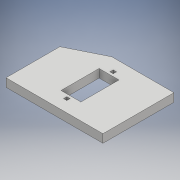
# Autodesk Inventor part: BackHand
Saved by Autodesk Inventor 2018 (Build 220112000, 112)
## iProperties
Created: 2018-02-14
Part Number: BackHand
Material: Générique
Document SubType Name: Modeling
Designer: Thomas
Density: 1 g/cm^3
Appearance: Par défaut
Author: Thomas
Autodesk Inventor part; units mm, degrees
ref_plane "YZ Plane" through (0, 0, 0) normal (1, 0, 0) x (0, 1, 0)
ref_plane "XZ Plane" through (0, 0, 0) normal (0, 1, 0) x (-1, 0, 0)
ref_plane "XY Plane" through (0, 0, 0) normal (0, 0, 1) x (1, 0, 0)
sketch "Esquisse1" plane through (0, 0, 0) normal (0, 0, 1) x (1, 0, 0)
  line L0 (0, 0) -> (0, 32.5)
  line L1 (0, 0) -> (58.5, 0)
  line L2 (58.5, 0) -> (58.5, 42.9)
  line L3 (58.5, 42.9) -> (21, 42.9)
  line L4 (0, 32.5) -> (21, 42.9)
  line L5 (58.5, 42.9) -> (0, 42.9) construction
  line L6 (0, 42.9) -> (0, 0) construction
  line L7 (0, 42.9) -> (58.5, 0) construction
  line L8 (58.5, 42.9) -> (0, 0) construction
  dimension "d0" = 32.5
  dimension "d1" = 58.5
  dimension "d2" = 42.9
  dimension "d3" = 37.5
  constraints: 18 end point, 3 horizontal, 2 vertical, 1 perpendicular
  measures "d0" distance of L0.start L0.end
  measures "d1" distance of L0.start L1.end
  measures "d2" distance of L1.end L2.end
  measures "d3" distance of L2.end L3.end
extrude "Extrusion1" add sketch "Esquisse1" along normal blind 5
sketch "Esquisse2" plane through (0, 0, 5) normal (0, 0, 1) x (1, 0, 0)
  line L0 (23.25, 32.95) -> (35.25, 32.95)
  line L1 (35.25, 32.95) -> (35.25, 9.95)
  line L2 (35.25, 9.95) -> (23.25, 9.95)
  line L3 (23.25, 9.95) -> (23.25, 32.95)
  line L4 (0, 32.5) -> (0, 0) projected
  line L5 (58.5, 42.9) -> (21, 42.9) projected
  line L6 (28.25, 36.45) -> (30.25, 36.45)
  line L7 (30.25, 36.45) -> (30.25, 34.45)
  line L8 (30.25, 34.45) -> (28.25, 34.45)
  line L9 (28.25, 34.45) -> (28.25, 36.45)
  line L10 (28.25, 8.45) -> (30.25, 8.45)
  line L11 (30.25, 8.45) -> (30.25, 6.45)
  line L12 (30.25, 6.45) -> (28.25, 6.45)
  line L13 (28.25, 6.45) -> (28.25, 8.45)
  dimension "d6" = 23
  dimension "d7" = 12
  dimension "d8" = 23.25
  dimension "d9" = 9.95
  dimension "d10" = 2
  dimension "d11" = 2
  dimension "d12" = 2
  dimension "d13" = 2
  dimension "d14" = 1.5
  dimension "d15" = 1.5
  dimension "d16" = 5
  dimension "d17" = 5
  constraints: 24 end point, 6 parallel, 3 horizontal, 3 perpendicular
  measures "d6" distance of L0.end L1.end
  measures "d7" distance of L1.end L2.end
  measures "d8" distance between parallel lines of L4 L3
  measures "d9" distance between parallel lines of L5 L0
  measures "d10" distance of L8.end L6.start
  measures "d11" distance of L7.end L8.end
  measures "d12" distance of L10.end L11.end
  measures "d13" distance of L10.start L10.end
  measures "d14" distance between parallel lines of L0 L8
  measures "d15" distance between parallel lines of L2 L10
  measures "d16" distance between parallel lines of L13 L3
  measures "d17" distance between parallel lines of L3 L9
extrude "Extrusion2" cut sketch "Esquisse2" against normal blind 5
